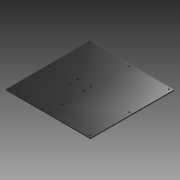
# Autodesk Inventor part: EnclosurePanelRight
Saved by Autodesk Inventor 2015 SP1 (Build 190203100, 203)
## iProperties
Category: Panel
Created: 2015-01-12
Part Number: EnclosurePanelRight
Material: ABS Plastic
Document SubType Name: Modeling
Designer: Jack
Density: 1.06 g/cm^3
Appearance: Smooth - Dark Gray
Mass: 893.587 g
Surface Area: 3634.87 cm^2
Volume: 843.007 cm^3
Vendor: Tap Plastics
Catalog Web Link: N/A
Author: Jack
Title: Enclosure Panel Right
Autodesk Inventor part; units mm, degrees
ref_plane "YZ Plane" through (0, 0, 0) normal (1, 0, 0) x (0, 1, 0)
ref_plane "XZ Plane" through (0, 0, 0) normal (0, 1, 0) x (-1, 0, 0)
ref_plane "XY Plane" through (0, 0, 0) normal (0, 0, 1) x (1, 0, 0)
sketch "Sketch1" plane through (0, 0, 0) normal (0, 0, 1) x (1, 0, 0)
  line L0 (0, 0) -> (424.7625, 0)
  line L1 (424.7625, 0) -> (424.7625, 420)
  line L2 (424.7625, 420) -> (0, 420)
  line L3 (0, 420) -> (0, 0)
  dimension "d0" = 424.7625
  dimension "d1" = 420
  constraints: 8 end point, 2 parallel, 1 horizontal, 1 perpendicular
  measures "d0" distance of L2.end L1.end
  measures "d1" distance of L0.end L1.end
extrude "Extrusion1" add sketch "Sketch1" along normal blind 4.7625
sketch "Sketch6" plane through (0, 0, 4.7625) normal (0, 0, 1) x (1, 0, 0)
  line L0 (0, 0) -> (424.7625, 0) projected
  line L1 (424.7625, 0) -> (424.7625, 420) projected
  line L2 (424.7625, 420) -> (0, 420) projected
  line L3 (0, 420) -> (0, 0) projected
  circle A0 centre (10, 410) radius 2.25
  circle A1 centre (410, 410) radius 2.25
  circle A2 centre (10, 10) radius 2.25
  circle A3 centre (410, 10) radius 2.25
  circle A4 centre (10, 210) radius 2.25
  circle A5 centre (410, 210) radius 2.25
  circle A6 centre (209.8815, 410) radius 2.25
  circle A7 centre (209.8815, 10) radius 2.25
  circle A8 centre (209.8815, 75) radius 2.25
  dimension "d42" = 4.5
  dimension "d43" = 10
  dimension "d44" = 10
  dimension "d45" = 14.7625
  dimension "d46" = 10
  dimension "d47" = 10
  dimension "d48" = 210
  dimension "d51" = 209.8815
  dimension "d55" = 75
  constraints: 9 centre point, 8 equal radius, 6 vertical alignment, 4 horizontal alignment
  measures "d42" diameter of A0
  measures "d43" distance from line of L2 A0.centre
  measures "d44" distance from line of L3 A0.centre
  measures "d45" distance from line of L1 A1.centre
  measures "d46" distance from line of L2 A1.centre
  measures "d47" distance from line of L0 A2.centre
  measures "d48" distance from line of L0 A5.centre
  measures "d51" distance from line of L3 A6.centre
  measures "d55" distance from line of L0 A8.centre
extrude "Extrusion3" cut sketch "Sketch6" against normal up to next contours A0 | A1 | A2 | A3 | A4 | A5 | A6 | A7 | A8
chamfer "Chamfer1" distance 2 angle 45 9 edges at (7.75, 410, 4.7625) (207.6315, 410, 4.7625) (407.75, 410, 4.7625) (407.75, 210, 4.7625) (7.75, 210, 4.7625) (7.75, 10, 4.7625) (207.6315, 10, 4.7625) (407.75, 10, 4.7625) (207.6315, 75, 4.7625)
sketch "Sketch7" plane through (0, 0, 4.7625) normal (0, 0, 1) x (1, 0, 0)
  line L0 (0, 0) -> (424.7625, 0) projected
  line L1 (424.7625, 0) -> (424.7625, 420) projected
  line L2 (0, 420) -> (0, 0) projected
  line L3 (0, 180) -> (424.7625, 180) construction
  line L4 (424.7625, 420) -> (0, 420) construction
  line L5 (130, 420) -> (130, 0) construction
  line L6 (0, 0) -> (424.7625, 0) construction
  point P0 (137.5, 222.5)
  point P1 (202.5, 222.5)
  point P2 (137.5, 187.5)
  point P3 (202.5, 187.5)
  dimension "d56" = 130
  dimension "d57" = 180
  dimension "d58" = 7.5
  dimension "d59" = 7.5
  dimension "d60" = 35
  dimension "d61" = 65
  constraints: 4 end point, 4 point on line, 2 horizontal alignment, 2 perpendicular, 2 vertical alignment
  measures "d56" distance between parallel lines of L2 L5
  measures "d57" distance between parallel lines of L6 L3
  measures "d58" distance from line of L3 point (137.5, 187.5)
  measures "d59" distance from line of L5 point (137.5, 187.5)
  measures "d60" distance of point (137.5, 187.5) point (137.5, 222.5)
  measures "d61" distance of point (202.5, 222.5) point (137.5, 222.5)
hole "Hole3" at (137.5, 222.5, 4.7625) at (202.5, 222.5, 4.7625) at (137.5, 187.5, 4.7625) at (202.5, 187.5, 4.7625) direction (0, 0, -1) diameter 4.5 end through all countersink diameter 8.5 countersink angle 90
body "Solid1"
